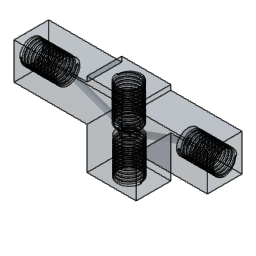
pH_sensor_incline (Autodesk Fusion 360 design; units mm, degrees)
Autodesk Fusion 360 part; units mm, degrees
sketch "Skizze1" plane through (0, 0, 0) normal (1, 0, 0) x (0, 1, 0)
  line L0 (-25, 16.0337) -> (0, 16.0337)
  line L1 (0, 16.0337) -> (0, -25)
  line L2 (0, -25) -> (-25, -25)
  line L3 (-25, -25) -> (-25, 16.0337)
  constraint horizontal L0
  constraint vertical L1
  constraint horizontal L2
  constraint vertical L3
extrude "Extrusion1" add sketch "Skizze1" along normal blind 30.3 makes body 1
move_body "Verschieben1" bodies 1 to x (0, 0, 1) y (0, 1, 0) z (-1, 0, 0) at (-25, 0, -25)
sketch "Skizze3" plane through (0, 0, 0) normal (1, 0, 0) x (0, 1, 0)
  circle A0 centre (20, 5) radius 0.8
  dimension "d29" = 1.6
  measures "d29" diameter of A0
extrude "Extrusion2" add sketch "Skizze3" along normal blind 17 separate body makes body 2
move_body "Verschieben2" bodies 2 to x (0.866025, 0, -0.5) y (0, 1, 0) z (0.5, 0, 0.866025) at (10.7565, 0, 0.86)
move_body "Verschieben3" bodies 2 to x (1, 0, 0) y (0, 1, 0) z (0, 0, 1) at (-51.0328, -31.9974, -7.7783)
move_body "Verschieben4" bodies 2 to x (1, 0, 0) y (0, 1, 0) z (0, 0, 1) at (-21.3282, 0, 0)
move_body "Verschieben5" bodies 2 to x (1, 0, 0) y (0, 1, 0) z (0, 0, 1) at (14.4979, 0.494, 25.1111)
move_body "Verschieben6" bodies 2 to x (1, 0, 0) y (0, 1, 0) z (0, 0, 1) at (6.968, -1.1918, -24.9313)
move_body "Verschieben7" bodies 2 to x (1, 0, 0) y (0, 1, 0) z (0, 0, 1) at (0.1918, 0, 0.1279)
copy_body "Körper kopieren/einfügen2" bodies 2 makes body 3
move_body "Verschieben8" bodies 3 to x (-0.5, 0, -0.866025) y (0, 1, 0) z (0.866025, 0, -0.5) at (-35.8241, 0, -48.4694)
move_body "Verschieben9" bodies 3 to x (1, 0, 0) y (0, 1, 0) z (0, 0, 1) at (15.5341, 0, 12.5935)
sketch "Skizze5" plane through (0, 0, 0) normal (1, 0, 0) x (0, 1, 0)
  circle A0 centre (11.614, 3.6415) radius 3.1
  dimension "d47" = 6.2
  measures "d47" diameter of A0
extrude "Extrusion3" add sketch "Skizze5" along normal blind 14.3 separate body makes body 4
sketch "Skizze6" plane through (14.3, 0, 0) normal (1, 0, 0) x (0, 1, 0)
  circle A0 centre (11.614, 3.6415) radius 3.1
  circle A1 centre (11.614, 3.6415) radius 2
  dimension "d50" = 4
  constraint concentric A0 A1
  measures "d50" diameter of A1
extrude "Extrusion4" add sketch "Skizze6" along normal blind 2 contours A1 bodies 4
fillet "Abrundung1" radius 2 1 faces at (16.3, 12.2368, 3.2551) on bodies 4
move_body "Verschieben10" bodies 4 to x (0, 0, 1) y (0, 1, 0) z (-1, 0, 0) at (0.5415, 0, 0.5415)
move_body "Verschieben11" bodies 4 to x (1, 0, 0) y (0, 1, 0) z (0, 0, 1) at (-17.5, 0, -29)
move_body "Verschieben12" bodies 4 to x (1, 0, 0) y (0, 1, 0) z (0, 0, 1) at (0, -24.5, 0)
move_body "Verschieben13" bodies 4 to x (1, 0, 0) y (0, 1, 0) z (0, 0, 1) at (0, 0, 1)
move_body "Verschieben14" bodies 4 to x (1, 0, 0) y (0, 1, 0) z (0, 0, 1) at (0, 0.2, 0)
move_body "Verschieben15" bodies 4 to x (-1, 0, 0) y (0, 1, 0) z (0, 0, -1) at (-40.9, 0, -16.917)
move_body "Verschieben16" bodies 4 to x (1, 0, 0) y (0, 1, 0) z (0, 0, 1) at (0, 0, -4)
sketch "Skizze7" plane through (0, 0, 0) normal (0, 0, 1) x (1, 0, 0)
  circle A0 centre (5, 10) radius 3
  dimension "d55" = 6
  measures "d55" diameter of A0
extrude "Extrusion5" add sketch "Skizze7" along normal blind 14.3 separate body makes body 5
sketch "Skizze8" plane through (0, 0, 14.3) normal (0, 0, 1) x (-1, 0, 0)
  circle A0 centre (-5, -10) radius 3
  circle A1 centre (-5, -10) radius 2
  dimension "d58" = 4
  constraint concentric A0 A1
  measures "d58" diameter of A1
extrude "Extrusion6" add sketch "Skizze8" along normal blind 0.5 contours A1 bodies 5
move_body "Verschieben17" bodies 5 to x (1, 0, 0) y (0, 1, 0) z (0, 0, 1) at (-25.5, 12, -27)
move_body "Verschieben18" bodies 5 to x (1, 0, 0) y (0, 1, 0) z (0, 0, 1) at (0, -34.5, 0)
move_body "Ausrichten1" bodies 5 to x (1, 0, 0) y (0, 1, 0) z (0, 0, 1) at (0.2, -0.186, 0)
move_body "Verschieben19" bodies 4 to x (1, 0, 0) y (0, 1, 0) z (0, 0, 1) at (0, 0, -1)
move_body "Verschieben20" bodies 4 to x (1, 0, 0) y (0, 1, 0) z (0, 0, 1) at (-0.2, 0, 0)
move_body "Verschieben21" bodies 5 to x (1, 0, 0) y (0, 1, 0) z (0, 0, 1) at (0, 0, 0.5)
move_body "Verschieben22" bodies 5 to x (1, 0, 0) y (0, 1, 0) z (0, 0, 1) at (-0.2, 0, 0)
move_body "Verschieben23" bodies 5 to x (1, 0, 0) y (0, 1, 0) z (0, 0, 1) at (0, 0, -3)
move_body "Verschieben24" bodies 4 to x (1, 0, 0) y (0, 1, 0) z (0, 0, 1) at (0, 0, 2)
sketch "Skizze9" plane through (0, 0, 0) normal (1, 0, 0) x (0, 1, 0)
  circle A0 centre (6.6918, 7.4769) radius 0.8
  dimension "d61" = 1.6
  measures "d61" diameter of A0
move_body "Verschieben34" bodies 5 to x (1, 0, 0) y (0, 1, 0) z (0, 0, 1) at (0, 0, 3.5)
move_body "Verschieben35" bodies 4 to x (1, 0, 0) y (0, 1, 0) z (0, 0, 1) at (0, 0, -1.9)
move_body "Verschieben36" bodies 2 to x (0.984808, 0, 0.173648) y (0, 1, 0) z (-0.173648, 0, 0.984808) at (-1.356, 0, 4.1293)
move_body "Verschieben37" bodies 3 to x (0.984808, 0, -0.173648) y (0, 1, 0) z (0.173648, 0, 0.984808) at (1.7131, 0, -3.4157)
move_body "Verschieben38" bodies 3 to x (1, 0, 0) y (0, 1, 0) z (0, 0, 1) at (-0.8508, -0.0215, 0.3864)
move_body "Verschieben40" bodies 2 to x (1, 0, 0) y (0, 1, 0) z (0, 0, 1) at (0, 0, -0.1)
move_body "Ausrichten2" bodies 2 to x (1, 0, 0) y (0, 1, 0) z (0, 0, 1) at (18.8373, -0.0215, 0.0344)
move_body "Verschieben41" bodies 2 to x (1, 0, 0) y (0, 1, 0) z (0, 0, 1) at (-18.5, 0, 0)
hole "Bohrung14" at (0, -12.7075, -4.998) direction (-1, 0, 0) diameter 6.5 depth 4 tip angle 180 bodies 1 3
hole "Bohrung15" at (-41.0337, -12.6821, -5.0324) direction (1, 0, 0) diameter 6.5 depth 4 tip angle 180 bodies 1 2
move_body "Verschieben49" bodies 4 to x (1, 0, 0) y (0, 1, 0) z (0, 0, 1) at (0.3, 0, 0)
move_body "Verschieben50" bodies 5 to x (1, 0, 0) y (0, 1, 0) z (0, 0, 1) at (0.3, 0, 0)
sketch "Skizze10" plane through (0, 0, 0) normal (1, 0, 0) x (0, 1, 0)
  circle A0 centre (21, 5) radius 0.8
  dimension "d70" = 1.6
  measures "d70" diameter of A0
move_body "Verschieben58" bodies 2 3 to x (1, 0, 0) y (0, 1, 0) z (0, 0, 1) at (-35, 0, 0)
loft "Erhebung1" add section 1 face at (-53.8327, -12.9094, -10.9605) section 2 face at (-56.41, -12.5212, -10.181) on bodies 2 3 bodies 3 2
move_body "Verschieben59" bodies 3 to x (1, 0, 0) y (0, 1, 0) z (0, 0, 1) at (35, 0, 0)
move_body "Verschieben60" bodies 5 to x (1, 0, 0) y (0, 1, 0) z (0, 0, 1) at (0, 0, 0.1)
combine "Kombinieren1" operation cut target body 1 tool bodies 3 4 5
extrude "Extrusion9" cut 1 faces at (-13.6779, -25, -14.9) along direction (0, 1, 0) blind 7.5 on bodies 1 bodies 1
extrude "Extrusion10" cut 1 faces at (-27.3558, 0, -14.9) along direction (0, -1, 0) blind 7.5 on bodies 1 bodies 1
box "Grundkörper Quader1" cut length 13 width 17 height -13 placed x (0, 0, 1) y (1, 0, 0) z (0, 1, 0) at (-44, -7.5, -25) bodies 1
box "Grundkörper Quader2" cut length 13 width 13 height -10 placed x (0, 0, -1) y (-1, 0, 0) z (0, 1, 0) at (0, -7.5, -12) bodies 1
box "Grundkörper Quader3" cut length 12.9499 width 0.5213 height -13 placed x (0, 0, -1) y (-1, 0, 0) z (0, 1, 0) at (-13, -7.5, -12.0501) bodies 1
delete_face "Fläche löschen1" 2 faces at (-13, -14.1667, -12.0334) (-13.1738, -14.1667, -12.0501) on bodies 1
box "Grundkörper Quader4" cut length 5.3 width 14.0337 height -13 placed x (0, 0, -1) y (1, 0, 0) z (0, -1, 0) at (-41.0337, -17.5, 5.3) bodies 1
box "Grundkörper Quader5" cut length 5.2559 width 13.5213 height -19 placed x (0, 0, 1) y (-1, 0, 0) z (0, -1, 0) at (0, -17.5, 0.0441) bodies 1
extrude "Extrusion11" cut 1 faces at (-18.0142, -7.5, -20.6667) along direction (0, -1, 0) blind 0.5 on bodies 1 bodies 1
move_body "Verschieben61" bodies 1 to x (1, 0, 0) y (0, 1, 0) z (0, 0, 1) at (0, 12.5527, 20.0069)
move_body "Verschieben62" bodies 1 to x (1, 0, 0) y (0, 1, 0) z (0, 0, 1) at (0, 0.1535, 0)
hole "Bohrung16" at (-20.2, 0.0202, -4.9931) direction (0, 0, 1) diameter 6.2 depth 13.4 tip angle 180 bodies 1
extrude "Extrusion12" add 1 faces at (0, -0.0296, 9.2576) along direction (1, 0, 0) blind 10 on bodies 1 bodies 1
extrude "Extrusion13" add 1 faces at (-41.0337, -0.0211, 9.2461) along direction (-1, 0, 0) blind 10 on bodies 1 bodies 1
extrude "Extrusion14" cut 1 faces at (-25.7638, -0.0996, 25.3069) along direction (0, 0, -1) blind 1.4 on bodies 1 bodies 1
extrude "Extrusion15" cut 1 faces at (-25.7638, -0.0996, -4.9931) along direction (0, 0, 1) blind 0.5 on bodies 1 bodies 1
extrude "Extrusion16" cut 1 faces at (-25.7638, -0.0996, -4.4931) along direction (0, 0, 1) blind 3 on bodies 1 bodies 1
extrude "Extrusion17" cut 1 faces at (-25.7638, -0.0996, 23.9069) along direction (0, 0, -1) blind 2.5 on bodies 1 bodies 1
hole "Bohrung17" at (-20.2794, -0.0635, 21.4069) direction (0, 0, -1) diameter 6.5 depth 10 tip angle 180 bodies 1
hole "Bohrung18" at (-20.2, 0.0202, -1.4931) direction (0, 0, 1) diameter 6.5 depth 10 tip angle 180 bodies 1
box "Grundkörper Quader6" cut length 1.8955 width 23.5213 height -12 placed x (0, 0, 1) y (-1, 0, 0) z (0, -1, 0) at (10, -4.7938, 8.0069) bodies 1
box "Grundkörper Quader7" cut length 1.95 width 24.0337 height -10 placed x (0, 0, -1) y (1, 0, 0) z (0, -1, 0) at (-51.0337, -4.7938, 9.9569) bodies 1
extrude "Extrusion18" cut 1 faces at (10, -0.0296, 10.5212) along direction (-1, 0, 0) blind 4 on bodies 1 bodies 1
extrude "Extrusion19" cut 1 faces at (-51.0337, -0.0211, 19.4128) along direction (1, 0, 0) blind 4 on bodies 1 bodies 1
coil "Grundkörper Spirale3" add diameter 6.5 section triangle in size 0.4 inside turns 10.5 pitch 0.9 right hand placed x (0, 1, 0) y (0, 0, -1) z (-1, 0, 0) at (6, -0.0013, 15.0089) bodies 1
delete_face "Fläche löschen2" 1 faces at (6.1474, 3.2453, 14.8601) on bodies 1
coil "Grundkörper Spirale5" add diameter 6.5 section triangle in size 0.4 inside turns 10.5 pitch 0.9 right hand placed x (0, -1, 0) y (0, 0, -1) z (1, 0, 0) at (-47.0337, 0.0241, 14.9745) bodies 1
delete_face "Fläche löschen4" 1 faces at (-47.1811, -3.2225, 14.8257) on bodies 1
coil "Grundkörper Spirale6" add diameter 6.5 section triangle in size 0.4 inside turns 10.5 pitch 0.9 right hand placed x (-1, 0, 0) y (0, 1, 0) z (0, 0, -1) at (-20.2794, -0.0635, 21.4069) bodies 1
coil "Grundkörper Spirale7" add diameter 6.5 section triangle in size 0.4 inside turns 10.5 pitch 0.9 right hand placed x (1, 0, 0) y (0, 1, 0) z (0, 0, 1) at (-20.2, 0.0202, -1.4931) bodies 1
delete_face "Fläche löschen5" 1 faces at (-16.9534, 0.169, -1.6405) on bodies 1
delete_face "Fläche löschen6" 1 faces at (-23.5259, 0.0858, 21.5543) on bodies 1
sketch "Skizze31" plane through (0, 0, 0) normal (0, 0, 1) x (1, 0, 0)
  circle A0 centre (12, 3) radius 2.15
  dimension "d179" = 4.3
  measures "d179" diameter of A0
extrude "Extrusion21" add sketch "Skizze31" along normal blind 2 separate body makes body 6
fillet "Abrundung3" radius 2 1 faces at (11.4746, 2.7262, 2) on bodies 6
move_body "Verschieben65" bodies 6 to x (-1, 0, 0) y (0, 1, 0) z (0, 0, -1) at (24, 0, -0.2)
move_body "Verschieben66" bodies 6 to x (1, 0, 0) y (0, 1, 0) z (0, 0, 1) at (-32.2, -2.99, 11.6)
combine "Kombinieren2" operation cut target body 1 tool bodies 6
sketch "Skizze32" plane through (0, 0, 0) normal (0, 0, 1) x (1, 0, 0)
  circle A0 centre (12.6428, 8.3666) radius 2.15
  dimension "d184" = 4.3
  measures "d184" diameter of A0
extrude "Extrusion22" add sketch "Skizze32" along normal blind 0.6 separate body makes body 7
move_body "Verschieben67" bodies 7 to x (1, 0, 0) y (0, 1, 0) z (0, 0, 1) at (-32.85, 0, 8.31)
combine "Kombinieren3" operation cut target body 1 tool bodies 7
